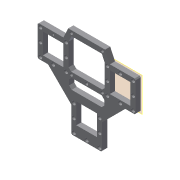
# Autodesk Inventor part: cellSTORM_inverted_base_vß
Saved by Autodesk Inventor 2019.4 (Build 234330000, 330)
## iProperties
Created: 2020-11-05
Part Number: cellSTORM_inverted_base_vß
Material: Generic
Document SubType Name: Modeling
Designer: diederichbenedict
Density: 1 g/cm^3
Appearance: Default
Author: diederichbenedict
Autodesk Inventor part; units mm, degrees
ref_plane "YZ Plane" through (0, 0, 0) normal (1, 0, 0) x (0, 1, 0)
ref_plane "XZ Plane" through (0, 0, 0) normal (0, 1, 0) x (-1, 0, 0)
ref_plane "XY Plane" through (0, 0, 0) normal (0, 0, 1) x (1, 0, 0)
ref_plane "Work Plane1" through (0, 0, 0) normal (0, 0, 1) x (1, 0, 0)
sketch "Sketch1" plane through (0, 0, 0) normal (0, 0, 1) x (1, 0, 0)
  circle A0 centre (0, 25) radius 1.95 projected
  circle A1 centre (-25, 0) radius 1.95 projected
  circle A2 centre (-25, -25) radius 1.95 projected
  circle A3 centre (25, 25) radius 1.95 projected
  circle A4 centre (25, -25) radius 1.95 projected
  circle A5 centre (-25, 25) radius 1.95 projected
  circle A6 centre (25, 0) radius 1.95 projected
  circle A7 centre (0, -25) radius 1.95 projected
  line L0 (-28, 30) -> (-30, 28) projected
  line L1 (-30, 28) -> (-30, -28) projected
  line L2 (-30, -28) -> (-28, -30) projected
  line L3 (-28, -30) -> (28, -30) projected
  line L4 (28, -30) -> (30, -28) projected
  line L5 (30, -28) -> (30, 28) projected
  line L6 (30, 28) -> (28, 30) projected
  line L7 (28, 30) -> (-28, 30) projected
  circle A8 centre (-130, 25) radius 1.95 projected
  circle A9 centre (-105, 0) radius 1.95 projected
  circle A10 centre (-105, -25) radius 1.95 projected
  circle A11 centre (-155, 25) radius 1.95 projected
  circle A12 centre (-155, -25) radius 1.95 projected
  circle A13 centre (-105, 25) radius 1.95 projected
  circle A14 centre (-155, 0) radius 1.95 projected
  circle A15 centre (-130, -25) radius 1.95 projected
  line L8 (-102, 30) -> (-100, 28) projected
  line L9 (-100, 28) -> (-100, -28) projected
  line L10 (-100, -28) -> (-102, -30) projected
  line L11 (-102, -30) -> (-158, -30) projected
  line L12 (-158, -30) -> (-160, -28) projected
  line L13 (-160, -28) -> (-160, 28) projected
  line L14 (-160, 28) -> (-158, 30) projected
  line L15 (-158, 30) -> (-102, 30) projected
  circle A16 centre (-90, -95) radius 1.95 projected
  circle A17 centre (-65, -70) radius 1.95 projected
  circle A18 centre (-40, -70) radius 1.95 projected
  circle A19 centre (-90, -120) radius 1.95 projected
  circle A20 centre (-40, -120) radius 1.95 projected
  circle A21 centre (-90, -70) radius 1.95 projected
  circle A22 centre (-65, -120) radius 1.95 projected
  circle A23 centre (-40, -95) radius 1.95 projected
  line L16 (-95, -67) -> (-93, -65) projected
  line L17 (-93, -65) -> (-37, -65) projected
  line L18 (-37, -65) -> (-35, -67) projected
  line L19 (-35, -67) -> (-35, -123) projected
  line L20 (-35, -123) -> (-37, -125) projected
  line L21 (-37, -125) -> (-93, -125) projected
  line L22 (-93, -125) -> (-95, -123) projected
  line L23 (-95, -123) -> (-95, -67) projected
  line L24 (-100, -20) -> (-30, -20)
  line L25 (-35, -75) -> (10, -30)
  line L26 (-35, -75) -> (28.6396, -75) construction
  line L27 (-95, -75) -> (-140, -30)
  line L28 (-45, -65) -> (-85, -65)
  line L29 (-85, -65) -> (-85, -105)
  line L30 (-85, -105) -> (-45, -105)
  line L31 (-45, -105) -> (-45, -65)
  line L32 (-45, -65) -> (-85, -105) construction
  line L33 (-85, -65) -> (-45, -105) construction
  line L34 (-110, 20) -> (-150, 20)
  line L35 (-150, 20) -> (-150, -20)
  line L36 (-150, -20) -> (-110, -20)
  line L37 (-110, -20) -> (-110, 20)
  line L38 (-110, 20) -> (-150, -20) construction
  line L39 (-150, 20) -> (-110, -20) construction
  line L40 (20, 20) -> (-20, 20)
  line L41 (-20, 20) -> (-20, -20)
  line L42 (-20, -20) -> (20, -20)
  line L43 (20, -20) -> (20, 20)
  line L44 (20, 20) -> (-20, -20) construction
  line L45 (-20, 20) -> (20, -20) construction
  point P0 (0, 0)
  point P1 (-65, -85)
  point P2 (-130, 0)
  dimension "d0" = 45
  dimension "d1" = 10
  dimension "d2" = 20
  dimension "d3" = 20
  dimension "d4" = 135
  dimension "d5" = 40
  dimension "d6" = 40
  dimension "d7" = 40
  dimension "d8" = 40
  dimension "d9" = 40
  dimension "d10" = 40
  constraints: 44 end point, 6 midpoint, 6 parallel, 6 point on line, 4 horizontal, 4 perpendicular, 1 equal length
  measures "d0" angle of L26 L25
  measures "d1" distance between parallel lines of L3 L24
  measures "d2" distance from line of L5 L25.end
  measures "d3" distance from line of L13 L27.end
  measures "d4" angle of L23 L27
  measures "d5" distance of L30.end L29.end
  measures "d6" distance of L29.end L28.end
  measures "d7" distance of L36.end L35.end
  measures "d8" distance of L35.end L34.end
  measures "d9" distance of L42.end L41.end
  measures "d10" distance of L41.end L40.end
extrude "Extrusion1" add sketch "Sketch1" along normal blind 10 contours L7 L6 L5 L4 L3 L2 L1 L0 | L1 L2 L3 L25 L19 L18 L17 L16 L23 L27 L11 L10 L9 L24 | L9 L10 L11 L12 L13 L14 L15 L8 | L19 L20 L21 L22 L23 L16 L17 L29 L30 L31 L18
sketch "Sketch2" plane through (0, 0, 10) normal (0, 0, 1) x (1, 0, 0)
  line L0 (-45, -65) -> (-45, -105) projected
  line L1 (-45, -105) -> (-85, -105) projected
  line L2 (-85, -105) -> (-85, -65) projected
  line L3 (-85, -65) -> (-45, -65) projected
  circle A0 centre (-40, -95) radius 1.95 projected
  circle A1 centre (-65, -120) radius 1.95 projected
  circle A2 centre (-90, -70) radius 1.95 projected
  circle A3 centre (-40, -120) radius 1.95 projected
  circle A4 centre (-90, -120) radius 1.95 projected
  circle A5 centre (-40, -70) radius 1.95 projected
  circle A6 centre (-90, -95) radius 1.95 projected
  line L4 (-110, 20) -> (-110, -20) projected
  line L5 (-110, -20) -> (-150, -20) projected
  line L6 (-150, -20) -> (-150, 20) projected
  line L7 (-150, 20) -> (-110, 20) projected
  circle A7 centre (-130, -25) radius 1.95 projected
  circle A8 centre (-155, 0) radius 1.95 projected
  circle A9 centre (-105, 25) radius 1.95 projected
  circle A10 centre (-155, -25) radius 1.95 projected
  circle A11 centre (-155, 25) radius 1.95 projected
  circle A12 centre (-105, -25) radius 1.95 projected
  circle A13 centre (-105, 0) radius 1.95 projected
  circle A14 centre (-130, 25) radius 1.95 projected
  line L8 (20, 20) -> (20, -20) projected
  line L9 (20, -20) -> (-20, -20) projected
  line L10 (-20, -20) -> (-20, 20) projected
  line L11 (-20, 20) -> (20, 20) projected
  circle A15 centre (0, -25) radius 1.95 projected
  circle A16 centre (25, 0) radius 1.95 projected
  circle A17 centre (-25, 25) radius 1.95 projected
  circle A18 centre (25, -25) radius 1.95 projected
  circle A19 centre (25, 25) radius 1.95 projected
  circle A20 centre (-25, -25) radius 1.95 projected
  circle A21 centre (-25, 0) radius 1.95 projected
  circle A22 centre (0, 25) radius 1.95 projected
  line L12 (-102, 30) -> (-158, 30) projected
  line L13 (-158, 30) -> (-160, 28) projected
  line L14 (-160, 28) -> (-160, -28) projected
  line L15 (-160, -28) -> (-158, -30) projected
  line L16 (-158, -30) -> (-140, -30) projected
  line L17 (-140, -30) -> (-95, -75) projected
  line L18 (-95, -75) -> (-95, -123) projected
  line L19 (-95, -123) -> (-93, -125) projected
  line L20 (-93, -125) -> (-37, -125) projected
  line L21 (-37, -125) -> (-35, -123) projected
  line L22 (-35, -123) -> (-35, -75) projected
  line L23 (-35, -75) -> (10, -30) projected
  line L24 (10, -30) -> (28, -30) projected
  line L25 (28, -30) -> (30, -28) projected
  line L26 (30, -28) -> (30, 28) projected
  line L27 (30, 28) -> (28, 30) projected
  line L28 (28, 30) -> (-28, 30) projected
  line L29 (-28, 30) -> (-30, 28) projected
  line L30 (-30, 28) -> (-30, -20) projected
  line L31 (-30, -20) -> (-100, -20) projected
  line L32 (-100, -20) -> (-100, 28) projected
  line L33 (-100, 28) -> (-102, 30) projected
  point P0 (0, 0)
hole "Hole1" at (-155, 25, 10) at (-155, 0, 10) at (-155, -25, 10) at (-130, -25, 10) at (-105, -25, 10) at (-105, 0, 10) at (-105, 25, 10) at (-25, 25, 10) at (-25, 0, 10) at (-25, -25, 10) at (0, -25, 10) at (25, -25, 10) at (25, 0, 10) at (25, 25, 10) at (0, 25, 10) at (-40, -70, 10) at (-90, -70, 10) at (-90, -95, 10) at (-90, -120, 10) at (-65, -120, 10) at (-40, -120, 10) at (-40, -95, 10) direction (0, 0, -1) diameter 4.5 depth 20 tip angle 118 counterbore diameter 7.5 counterbore depth 4
sketch "Sketch3" plane through (0, 0, 10) normal (0, 0, 1) x (1, 0, 0)
  circle A0 centre (-40, -120) radius 3.75 projected
  circle A1 centre (-90, -120) radius 3.75 projected
  circle A2 centre (-90, -70) radius 3.75 projected
  circle A3 centre (-40, -70) radius 3.75 projected
  circle A4 centre (25, 25) radius 3.75 projected
  circle A5 centre (25, -25) radius 3.75 projected
  circle A6 centre (-25, -25) radius 3.75 projected
  circle A7 centre (-25, 25) radius 3.75 projected
  circle A8 centre (-105, 0) radius 3.75 projected
  circle A9 centre (-130, -25) radius 3.75 projected
  circle A10 centre (-155, 0) radius 3.75 projected
  circle A11 centre (-155, 25) radius 3.75 projected
  circle A12 centre (-155, -25) radius 3.75 projected
  circle A13 centre (-105, -25) radius 3.75 projected
  circle A14 centre (-105, 25) radius 3.75 projected
  circle A15 centre (-25, 0) radius 3.75 projected
  circle A16 centre (0, -25) radius 3.75 projected
  circle A17 centre (25, 0) radius 3.75 projected
  circle A18 centre (0, 25) radius 3.75 projected
  circle A19 centre (-90, -95) radius 3.75 projected
  circle A20 centre (-65, -120) radius 3.75 projected
  circle A21 centre (-40, -95) radius 3.75 projected
  line L0 (-45, -65) -> (-45, -105) projected
  line L1 (-45, -105) -> (-85, -105) projected
  line L2 (-85, -105) -> (-85, -65) projected
  line L3 (-85, -65) -> (-45, -65) projected
  line L4 (-110, 20) -> (-110, -20) projected
  line L5 (-110, -20) -> (-150, -20) projected
  line L6 (-150, -20) -> (-150, 20) projected
  line L7 (-150, 20) -> (-110, 20) projected
  circle A22 centre (-130, 25) radius 1.95 projected
  line L8 (20, 20) -> (20, -20) projected
  line L9 (20, -20) -> (-20, -20) projected
  line L10 (-20, -20) -> (-20, 20) projected
  line L11 (-20, 20) -> (20, 20) projected
  line L12 (-102, 30) -> (-158, 30) projected
  line L13 (-158, 30) -> (-160, 28) projected
  line L14 (-160, 28) -> (-160, -28) projected
  line L15 (-160, -28) -> (-158, -30) projected
  line L16 (-158, -30) -> (-140, -30) projected
  line L17 (-140, -30) -> (-95, -75) projected
  line L18 (-95, -75) -> (-95, -123) projected
  line L19 (-95, -123) -> (-93, -125) projected
  line L20 (-93, -125) -> (-37, -125) projected
  line L21 (-37, -125) -> (-35, -123) projected
  line L22 (-35, -123) -> (-35, -75) projected
  line L23 (-35, -75) -> (10, -30) projected
  line L24 (10, -30) -> (28, -30) projected
  line L25 (28, -30) -> (30, -28) projected
  line L26 (30, -28) -> (30, 28) projected
  line L27 (30, 28) -> (28, 30) projected
  line L28 (28, 30) -> (-28, 30) projected
  line L29 (-28, 30) -> (-30, 28) projected
  line L30 (-30, 28) -> (-30, -20) projected
  line L31 (-30, -20) -> (-100, -20) projected
  line L32 (-100, -20) -> (-100, 28) projected
  line L33 (-100, 28) -> (-102, 30) projected
  line L34 (-99.1421, -30) -> (-30.8579, -30)
  line L35 (-30.8579, -30) -> (-20, -19.1421)
  line L36 (-20, -19.1421) -> (-20, 20)
  line L37 (-20, 20) -> (20, 20)
  line L38 (20, 20) -> (20, -20)
  line L39 (20, -20) -> (5.8579, -20)
  line L40 (5.8579, -20) -> (-45, -70.8579)
  line L41 (-45, -70.8579) -> (-45, -115)
  line L42 (-45, -115) -> (-85, -115)
  line L43 (-85, -115) -> (-85, -70.8579)
  line L44 (-85, -70.8579) -> (-135.8579, -20)
  line L45 (-135.8579, -20) -> (-150, -20)
  line L46 (-150, -20) -> (-150, 20)
  line L47 (-150, 20) -> (-110, 20)
  line L48 (-110, 20) -> (-110, -19.1421)
  line L49 (-110, -19.1421) -> (-99.1421, -30)
  line L50 (-99.1421, -30) -> (-30.8579, -30)
  line L51 (-30.8579, -30) -> (-30.8579, -50)
  line L52 (-30.8579, -50) -> (-99.1421, -50)
  line L53 (-99.1421, -50) -> (-99.1421, -30)
  point P0 (0, 0)
  dimension "d23" = 10
  dimension "d24" = 20
  constraints: 40 end point, 2 parallel, 1 horizontal, 1 perpendicular, 12 other
  measures "d23" distance between parallel lines of L31 L34
  measures "d24" distance of L50.end L51.end
extrude "Extrusion2" cut sketch "Sketch3" against normal through all contours L34 L51 L52 L53
chamfer "Chamfer2" distance 5 angle 45 6 edges at (-30.8579, -30, 5) (-30.8579, -50, 5) (-99.1421, -30, 5) (-99.1421, -50, 5) (-30, -20, 5) (-100, -20, 5)
sketch "Sketch4" plane through (0, 0, 10) normal (0, 0, 1) x (1, 0, 0)
  line L0 (-99.1421, -45) -> (-99.1421, -35) projected
  line L1 (-94.1421, -30) -> (-99.1421, -35) projected
  line L2 (-94.1421, -30) -> (-35.8579, -30) projected
  line L3 (-30.8579, -35) -> (-35.8579, -30) projected
  line L4 (-30.8579, -35) -> (-30.8579, -45) projected
  line L5 (-35.8579, -50) -> (-30.8579, -45) projected
  line L6 (-35.8579, -50) -> (-94.1421, -50) projected
  line L7 (-99.1421, -45) -> (-94.1421, -50) projected
  circle A0 centre (-40, -120) radius 3.75 projected
  circle A1 centre (-90, -120) radius 3.75 projected
  circle A2 centre (-90, -70) radius 3.75 projected
  circle A3 centre (0, 25) radius 3.75 projected
  circle A4 centre (25, 0) radius 3.75 projected
  circle A5 centre (0, -25) radius 3.75 projected
  circle A6 centre (-25, 0) radius 3.75 projected
  circle A7 centre (-105, 25) radius 3.75 projected
  circle A8 centre (-105, -25) radius 3.75 projected
  circle A9 centre (-155, -25) radius 3.75 projected
  circle A10 centre (-155, 25) radius 3.75 projected
  circle A11 centre (-155, 0) radius 3.75 projected
  circle A12 centre (-130, -25) radius 3.75 projected
  circle A13 centre (-105, 0) radius 3.75 projected
  circle A14 centre (-25, 25) radius 3.75 projected
  circle A15 centre (-25, -25) radius 3.75 projected
  circle A16 centre (25, -25) radius 3.75 projected
  circle A17 centre (25, 25) radius 3.75 projected
  circle A18 centre (-40, -70) radius 3.75 projected
  circle A19 centre (-90, -95) radius 3.75 projected
  circle A20 centre (-65, -120) radius 3.75 projected
  circle A21 centre (-40, -95) radius 3.75 projected
  line L8 (-45, -65) -> (-45, -105) projected
  line L9 (-45, -105) -> (-85, -105) projected
  line L10 (-85, -105) -> (-85, -65) projected
  line L11 (-85, -65) -> (-45, -65) projected
  line L12 (-110, 20) -> (-110, -20) projected
  line L13 (-110, -20) -> (-150, -20) projected
  line L14 (-150, -20) -> (-150, 20) projected
  line L15 (-150, 20) -> (-110, 20) projected
  circle A22 centre (-130, 25) radius 1.95 projected
  line L16 (20, 20) -> (20, -20) projected
  line L17 (20, -20) -> (-20, -20) projected
  line L18 (-20, -20) -> (-20, 20) projected
  line L19 (-20, 20) -> (20, 20) projected
  line L20 (-102, 30) -> (-158, 30) projected
  line L21 (-158, 30) -> (-160, 28) projected
  line L22 (-160, 28) -> (-160, -28) projected
  line L23 (-160, -28) -> (-158, -30) projected
  line L24 (-158, -30) -> (-140, -30) projected
  line L25 (-140, -30) -> (-95, -75) projected
  line L26 (-95, -75) -> (-95, -123) projected
  line L27 (-95, -123) -> (-93, -125) projected
  line L28 (-93, -125) -> (-37, -125) projected
  line L29 (-37, -125) -> (-35, -123) projected
  line L30 (-35, -123) -> (-35, -75) projected
  line L31 (-35, -75) -> (10, -30) projected
  line L32 (10, -30) -> (28, -30) projected
  line L33 (28, -30) -> (30, -28) projected
  line L34 (30, -28) -> (30, 28) projected
  line L35 (30, 28) -> (28, 30) projected
  line L36 (28, 30) -> (-28, 30) projected
  line L37 (-28, 30) -> (-30, 28) projected
  line L38 (-30, 28) -> (-30, -15) projected
  line L39 (-35, -20) -> (-30, -15) projected
  line L40 (-35, -20) -> (-95, -20) projected
  line L41 (-100, -15) -> (-95, -20) projected
  line L42 (-100, -15) -> (-100, 28) projected
  line L43 (-100, 28) -> (-102, 30) projected
  line L44 (-100.775, 50) -> (-29.225, 50)
  line L45 (-35.5957, 40) -> (-94.4043, 40)
  line L46 (-100.775, 50) -> (-110.1012, 30)
  line L47 (-100.775, 50) -> (-78.7075, 50) construction
  line L48 (-100, 28) -> (-102, 30) projected
  line L49 (-100, 28) -> (-94.4043, 40)
  line L50 (-29.225, 50) -> (-19.8988, 30)
  line L51 (28, 30) -> (-28, 30) projected
  line L52 (-29.225, 50) -> (-7.1574, 50) construction
  line L53 (-30, 28) -> (-35.5957, 40)
  line L54 (-30, 28) -> (-16.7595, 28) construction
  line L55 (28, 30) -> (-28, 30) projected
  point P0 (0, 0)
  dimension "deg_1" = 115
  dimension "d33" = 115
  dimension "d54" = 10
  dimension "d55" = 10
  dimension "d56" = 10
  dimension "d57" = 10
  constraints: 18 end point, 4 horizontal, 3 equal length, 3 parallel, 2 point on line
  measures "deg_1" angle of L46 L47
  measures "d33" angle of L54 L53
  measures "d54" distance between parallel lines of L44 L45
  measures "d55" distance between parallel lines of L49 L46
  measures "d56" distance between parallel lines of L50 L53
  measures "d57" distance between parallel lines of L45 L55
extrude "Extrusion3" add sketch "Sketch4" against normal up to surface (10 mm away) contours L20 L46 L44 L50 L36 L37 L53 L45 L49 L43
sketch "Sketch5" plane through (0, 0, 0) normal (0, 0, -1) x (-1, 0, 0)
  circle A0 centre (65, 12.1599) radius 7 projected
  line L0 (100.775, 50) -> (29.225, 50) projected
  line L1 (35.8579, -30) -> (94.1421, -30) projected
  circle A1 centre (95, -25) radius 3
  circle A2 centre (35, -25) radius 3
  circle A3 centre (35, 45) radius 3
  circle A4 centre (95, 45) radius 3
  line L2 (35, -20) -> (95, -20) projected
  circle A5 centre (65, -25) radius 3
  point P0 (0, 0)
  point P1 (65, -6.188)
  point P2 (101, 46)
  dimension "d38" = 6
  dimension "d39" = 6
  dimension "d40" = 6
  dimension "d43" = 5
  dimension "d44" = 6
  dimension "d45" = 5
  dimension "d48" = 5
  dimension "d49" = 5
  dimension "d51" = 6
  dimension "d59" = 30
  dimension "d60" = 30
  dimension "d61" = 0
  dimension "d62" = 0
  constraints: 5 centre point
  measures "d38" diameter of A1
  measures "d39" diameter of A2
  measures "d40" diameter of A3
  measures "d43" distance from line of A3.centre L0
  measures "d44" diameter of A4
  measures "d45" distance from line of A4.centre L0
  measures "d48" distance from line of L2 A2.centre
  measures "d49" distance from line of L2 A1.centre
  measures "d51" diameter of A5
  measures "d59" horizontal distance of A3.centre A0.centre
  measures "d60" horizontal distance of A4.centre A0.centre
  measures "d61" horizontal distance of A3.centre A2.centre
  measures "d62" horizontal distance of A4.centre A1.centre
extrude "Extrusion4" cut sketch "Sketch5" against normal through all
sketch "Sketch6" plane through (0, 0, 0) normal (0, 0, -1) x (-1, 0, 0)
  circle A0 centre (95, 45) radius 3 projected
  circle A1 centre (35, -25) radius 3 projected
  circle A2 centre (95, -25) radius 3 projected
  circle A3 centre (35, 45) radius 3 projected
  circle A4 centre (65, -25) radius 3 projected
  line L0 (100, -15) -> (100, 28) projected
  line L1 (95, -20) -> (100, -15) projected
  line L2 (35, -20) -> (95, -20) projected
  line L3 (30, -15) -> (35, -20) projected
  line L4 (30, 28) -> (30, -15) projected
  line L5 (30, 28) -> (35.5957, 40) projected
  line L6 (35.5957, 40) -> (94.4043, 40) projected
  line L7 (94.4043, 40) -> (100, 28) projected
  line L8 (99.1421, -35) -> (99.1421, -45) projected
  line L9 (94.1421, -50) -> (99.1421, -45) projected
  line L10 (94.1421, -50) -> (35.8579, -50) projected
  line L11 (30.8579, -45) -> (35.8579, -50) projected
  line L12 (30.8579, -45) -> (30.8579, -35) projected
  line L13 (35.8579, -30) -> (30.8579, -35) projected
  line L14 (35.8579, -30) -> (94.1421, -30) projected
  line L15 (99.1421, -35) -> (94.1421, -30) projected
  circle A5 centre (40, -120) radius 2.25 projected
  circle A6 centre (90, -120) radius 2.25 projected
  circle A7 centre (90, -70) radius 2.25 projected
  circle A8 centre (0, 25) radius 2.25 projected
  circle A9 centre (-25, 0) radius 2.25 projected
  circle A10 centre (0, -25) radius 2.25 projected
  circle A11 centre (25, 0) radius 2.25 projected
  circle A12 centre (105, 25) radius 2.25 projected
  circle A13 centre (105, -25) radius 2.25 projected
  circle A14 centre (155, -25) radius 2.25 projected
  circle A15 centre (155, 25) radius 2.25 projected
  circle A16 centre (155, 0) radius 2.25 projected
  circle A17 centre (130, -25) radius 2.25 projected
  circle A18 centre (105, 0) radius 2.25 projected
  circle A19 centre (25, 25) radius 2.25 projected
  circle A20 centre (25, -25) radius 2.25 projected
  circle A21 centre (-25, -25) radius 2.25 projected
  circle A22 centre (-25, 25) radius 2.25 projected
  circle A23 centre (40, -70) radius 2.25 projected
  circle A24 centre (90, -95) radius 2.25 projected
  circle A25 centre (65, -120) radius 2.25 projected
  circle A26 centre (40, -95) radius 2.25 projected
  line L16 (45, -105) -> (45, -65) projected
  line L17 (45, -65) -> (85, -65) projected
  line L18 (85, -65) -> (85, -105) projected
  line L19 (85, -105) -> (45, -105) projected
  line L20 (110, -20) -> (110, 20) projected
  line L21 (110, 20) -> (150, 20) projected
  line L22 (150, 20) -> (150, -20) projected
  line L23 (150, -20) -> (110, -20) projected
  circle A27 centre (130, 25) radius 1.95 projected
  line L24 (-20, -20) -> (-20, 20) projected
  line L25 (-20, 20) -> (20, 20) projected
  line L26 (20, 20) -> (20, -20) projected
  line L27 (20, -20) -> (-20, -20) projected
  line L28 (110.1012, 30) -> (100.775, 50) projected
  line L29 (100.775, 50) -> (29.225, 50) projected
  line L30 (29.225, 50) -> (19.8988, 30) projected
  line L31 (-28, 30) -> (19.8988, 30) projected
  line L32 (-30, 28) -> (-28, 30) projected
  line L33 (-30, -28) -> (-30, 28) projected
  line L34 (-28, -30) -> (-30, -28) projected
  line L35 (-10, -30) -> (-28, -30) projected
  line L36 (35, -75) -> (-10, -30) projected
  line L37 (35, -123) -> (35, -75) projected
  line L38 (37, -125) -> (35, -123) projected
  line L39 (93, -125) -> (37, -125) projected
  line L40 (95, -123) -> (93, -125) projected
  line L41 (95, -75) -> (95, -123) projected
  line L42 (140, -30) -> (95, -75) projected
  line L43 (158, -30) -> (140, -30) projected
  line L44 (160, -28) -> (158, -30) projected
  line L45 (160, 28) -> (160, -28) projected
  line L46 (158, 30) -> (160, 28) projected
  line L47 (110.1012, 30) -> (158, 30) projected
  line L48 (40.0564, 25.7619) -> (89.9436, 25.7619)
  line L49 (89.9436, 25.7619) -> (89.9436, 63.5954)
  line L50 (89.9436, 63.5954) -> (40.0564, 63.5954)
  line L51 (40.0564, 63.5954) -> (40.0564, 25.7619)
  line L52 (40.0564, 25.7619) -> (89.9436, 63.5954) construction
  line L53 (89.9436, 25.7619) -> (40.0564, 63.5954) construction
  point P0 (0, 0)
  point P1 (65, 44.6786)
  dimension "d63" = 0
  constraints: 12 end point, 2 midpoint, 2 parallel, 1 horizontal, 1 perpendicular
  measures "d63" horizontal distance of point (65, 44.679) A4.centre
extrude "Extrusion5" cut sketch "Sketch6" against normal through all contours L49 L48 L51 L6 | L6 L51 L29 L49 | L29 L51 L50 L49
equation "\"d33\" = deg_1"
body "Solid1"
